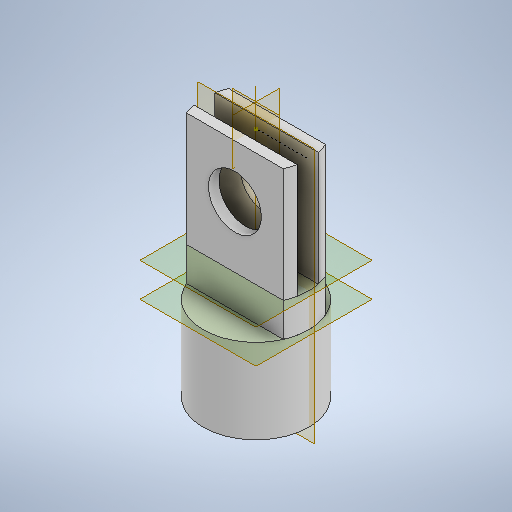
# Autodesk Inventor part: przegub
Saved by Autodesk Inventor 2025.2 (Build 292293000, 293)
## iProperties
Created: 2025-04-28
Part Number: przegub
Material: Ogólny
Document SubType Name: Modeling
Designer: marci
Density: 1 g/cm^3
Appearance: Domyślna
Author: marci
Autodesk Inventor part; units mm, degrees
ref_plane "YZ Plane" through (0, 0, 0) normal (1, 0, 0) x (0, 1, 0)
ref_plane "XZ Plane" through (0, 0, 0) normal (0, 1, 0) x (-1, 0, 0)
ref_plane "XY Plane" through (0, 0, 0) normal (0, 0, 1) x (1, 0, 0)
sketch "Szkic2" plane through (0, 0, 0) normal (0, 1, 0) x (-1, 0, 0)
  circle A0 centre (0, 0) radius 25
  line L0 (0, 0) -> (-25, 0)
  line L1 (0, 0) -> (25, 0)
  constraints: 4 end point, 2 horizontal, 2 point on circle, 1 centre point, 1 coincident
extrude "Wyciągnięcie proste1" add sketch "Szkic2" along normal blind 20 and the other way blind 50
sketch "Szkic3" plane through (0, 20, 0) normal (0, 1, 0) x (1, 0, 0)
  circle A0 centre (0, 0) radius 25 projected
  line L0 (0, 0) -> (0, -25)
  constraints: 2 end point, 1 vertical, 1 vertical alignment, 1 other
ref_plane "Płaszczyzna konstrukcyjna2" through (0, 20, 0) normal (0, 0, 1) x (1, 0, 0)
sketch "Szkic4" plane through (0, 20, 0) normal (0, 0, 1) x (1, 0, 0)
  circle A0 centre (0, -25) radius 12.5
  point P0 (0, -20)
  dimension "d6" = 25
  constraints: 1 centre point
  measures "d6" diameter of A0
extrude "Wyciągnięcie proste2" cut sketch "Szkic4" along normal through all both and the other way through all
sketch "Szkic5" plane through (0, 20, 0) normal (0, 0, 1) x (1, 0, 0)
  point P0 (0, -20)
sketch "Szkic6" plane through (0, 20, 0) normal (0, 1, 0) x (1, 0, 0)
  line L0 (0, 0) -> (24.7645, 0) construction
  constraints: 2 end point, 1 horizontal
ref_plane "Płaszczyzna konstrukcyjna3" through (0, 20, 0) normal (1, 0, 0) x (0, 1, 0)
ref_plane "Płaszczyzna konstrukcyjna4" through (0, -34, 0) normal (0, -1, 0) x (1, 0, 0)
split body "Podział3" result two bodies by plane through (0, -34, 0) normal (0, -1, 0) first body at (-24.1827, -39.3333, 3.9301)
sketch "Szkic9" plane through (0, 20, 0) normal (0, 1, 0) x (1, 0, 0)
  point P0 (0, 0)
sketch "Szkic10" plane through (0, 20, 0) normal (1, 0, 0) x (0, 1, 0)
  line L0 (0, -25) -> (0, 25) projected
  line L1 (-54, -25) -> (-54, 25) projected
  line L2 (0, 5) -> (-54, 5)
  line L3 (-54, 5) -> (-54, -5)
  line L4 (-54, -5) -> (0, -5)
  line L5 (0, -5) -> (0, 5)
  point P0 (-20, 0)
  dimension "d13" = 10
  constraints: 8 end point, 2 parallel, 2 point on line, 1 horizontal, 1 perpendicular
  measures "d13" distance of L3.end L2.end
extrude "Wyciągnięcie proste3" cut sketch "Szkic10" along normal through all both and the other way through all bodies 3
sketch "Szkic11" plane through (0, 20, 0) normal (1, 0, 0) x (0, 1, 0)
  line L0 (0, 10) -> (-55.9013, 10)
  line L1 (-55.9013, 10) -> (-55.9013, -10)
  line L2 (-55.9013, -10) -> (0, -10)
  line L3 (0, -10) -> (0, 10)
  point P0 (-20, 0)
  constraints: 8 end point, 2 parallel, 1 horizontal, 1 perpendicular
extrude "Wyciągnięcie proste4" cut sketch "Szkic11" along normal through all both and the other way through all keep common part bodies 3
ref_plane "Płaszczyzna konstrukcyjna5" through (0, -50, 0) normal (0, -1, 0) x (1, 0, 0)
extrude "Wyciągnięcie proste5" add sketch "Szkic3" against normal blind 40 from surface at -70 bodies 2
split body "Podział4" result two bodies by plane through (0, -50, 0) normal (0, -1, 0) bodies 2 first body at (24.4206, -76.6667, 1.9714)
ref_plane "Płaszczyzna konstrukcyjna6" through (-24.4949, 20, 0) normal (0, 0, 1) x (1, 0, 0)
sketch "Szkic13" plane through (0, -50, 0) normal (0, 1, 0) x (1, 0, 0)
  point P0 (0, 0)
sketch "Szkic14" plane through (-24.4949, 20, 0) normal (0, 0, 1) x (1, 0, 0)
  line L0 (-0.5051, -54) -> (49.4949, -54)
  line L1 (49.4949, -54) -> (49.4949, -70)
  line L2 (49.4949, -70) -> (-0.5051, -70)
  line L3 (-0.5051, -70) -> (-0.5051, -54)
  point P0 (24.4949, -20)
  constraints: 8 end point, 2 parallel, 1 horizontal, 1 perpendicular
extrude "Wyciągnięcie proste7" cut sketch "Szkic14" along normal mid plane 20 keep common part bodies 5
sketch "Szkic15" plane through (0, -90, 0) normal (0, -1, 0) x (1, 0, 0)
  point P0 (0, 0)
  point P1 (1.2927, -0.7334)
hole "Otwór1" at (1.2927, -90, -0.7334) direction (0, 1, 0) diameter 13.835 depth 41.3 tip angle 118 bodies 4 thread size "M16x2" class "6H" standard "ISO Metric profile"
